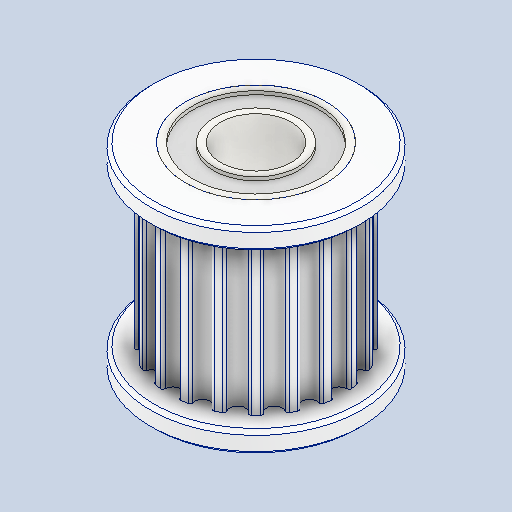
# Autodesk Inventor part: 9mm 20T GT2 Idler Pulley 5mm Bore
Saved by Autodesk Inventor 2024 (Build 280153000, 153)
## iProperties
Created: 2023-06-15
Part Number: 9mm 20T GT2 Idler Pulley 5mm Bore
Material: Aluminum 6061
Document SubType Name: Modeling
Designer: Ishaan
Density: 2.7 g/cm^3
Appearance: Aluminum - Flat
Author: Ishaan
Autodesk Inventor part; units mm, degrees
ref_plane "YZ Plane" through (0, 0, 0) normal (1, 0, 0) x (0, 1, 0)
ref_plane "XZ Plane" through (0, 0, 0) normal (0, 1, 0) x (-1, 0, 0)
ref_plane "XY Plane" through (0, 0, 0) normal (0, 0, 1) x (1, 0, 0)
sketch "Sketch1" plane through (0, 0, 0) normal (0, 0, 1) x (1, 0, 0)
  line L0 (0, 0) -> (-7.5, 0)
  line L1 (-7.5, 0) -> (-7.5, 1.5)
  line L2 (-7.5, 1.5) -> (0, 1.5)
  line L3 (0, 1.5) -> (0, 0)
  line L4 (0, 1.5) -> (-6.11, 1.5)
  line L5 (-6.11, 1.5) -> (-6.11, 12.5)
  line L6 (-6.11, 12.5) -> (0, 12.5)
  line L7 (0, 12.5) -> (0, 1.5)
  line L8 (0, 12.5) -> (-7.5, 12.5)
  line L9 (-7.5, 12.5) -> (-7.5, 14)
  line L10 (-7.5, 14) -> (0, 14)
  line L11 (0, 14) -> (0, 12.5)
  line L12 (0, 14) -> (-5, 14)
  line L13 (-5, 14) -> (-5, 0)
  line L14 (-5, 0) -> (0, 0)
  line L15 (0, 0) -> (0, 14)
  point P0 (-5, 14)
  point P1 (-6.11, 12.5)
  point P2 (-6.11, 1.5)
  dimension "d0" = 7.5
  dimension "d1" = 5
  dimension "d2" = 14
  dimension "d3" = 11
  dimension "d4" = 1.5
  dimension "d5" = 6.11
  constraints: 32 end point, 8 parallel, 4 horizontal, 4 perpendicular, 2 point on line
  measures "d0" distance between parallel lines of L3 L1
  measures "d1" distance between parallel lines of L13 L3
  measures "d2" distance between parallel lines of L0 L10
  measures "d3" distance between parallel lines of L2 L8
  measures "d4" distance between parallel lines of L0 L2
  measures "d5" distance between parallel lines of L7 L5
revolve "Revolution1" add sketch "Sketch1" angle 360 about axis through (0, 0, 0) along (0, 1, 0) contours L0 L1 L2 L13 | L2 L5 L6 L13 | L6 L8 L9 L10 L13
chamfer "Chamfer2" distance 0.25 angle 45 4 edges at (7.5, 12.5, 0) (7.5, 1.5, 0) (7.5, 0, 0) (7.5, 14, 0)
sketch "Sketch5" plane through (0, 12.5, 0) normal (0, -1, 0) x (1, 0, 0)
  circle A0 centre (0, 0) radius 6.11 projected
  circle A1 centre (0, 0) radius 5 projected
  circle A2 centre (0, 0) radius 6.11 construction
  circle A3 centre (0, 0) radius 6.11 construction
  arc A4 (-0.7227, -6.0671) -> (0.7227, -6.0671) centre (0, 0) ccw
  arc A5 (0.555, -5.9175) -> (0.7227, -6.0671) centre (0.705, -5.9182) ccw
  arc A6 (-0.7227, -6.0671) -> (-0.555, -5.9175) centre (-0.705, -5.9182) ccw
  arc A7 (0.555, -5.9175) -> (-0.555, -5.9175) centre (0, -5.915) ccw
  circle A8 centre (0, 0) radius 7.25 projected
  point P0 (0.7227, -6.0671)
  dimension "d22" = 12.22
  dimension "d23" = 0.15
  dimension "d24" = 0.555
  dimension "d25" = 0.75
  constraints: 8 point on circle, 5 centre point, 5 tangent, 1 coincident, 1 concentric, 1 equal radius, 1 vertical alignment
  measures "d22" diameter of A3
  measures "d23" radius of A5
  measures "d24" radius of A7
extrude "Extrusion2" cut sketch "Sketch5" along normal up to surface (11 mm away) contours A6 A7 A5 A0 picked at (-0.0224, -5.8582)
pattern_circular "Circular Pattern1" count 20 over 360 about axis through (0, 7, 0) along (0, 1, 0) of "Extrusion2"
ref_plane "Work Plane5" through (0, 12, 0) normal (0, 1, 0) x (1, 0, 0)
sketch "Sketch6" plane through (0, 12, 0) normal (0, 1, 0) x (1, 0, 0)
  circle A0 centre (0, 0) radius 5
  circle A1 centre (0, 0) radius 2.5
  circle A2 centre (0, 0) radius 4.5
  circle A3 centre (0, 0) radius 3
  dimension "d36" = 10
  dimension "d37" = 5
  dimension "d38" = 0.5
  dimension "d39" = 0.5
  constraints: 4 centre point, 2 coincident
  measures "d36" diameter of A0
  measures "d37" diameter of A1
  measures "d38" radial gap between concentric circles of A0 A2
  measures "d39" radial gap between concentric circles of A1 A3
extrude "Extrusion3" add sketch "Sketch6" along normal mid plane 4 separate body
extrude "Extrusion4" add sketch "Sketch6" along normal mid plane 3.5 contours A2 bodies 2
ref_plane "Work Plane4" through (0, 7, 0) normal (0, -1, 0) x (1, 0, 0)
mirror "Mirror3" about plane through (0, 7, 0) normal (0, -1, 0) bodies 2 separate body
body "Solid1"
